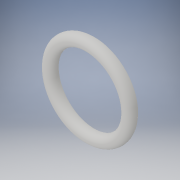
# Autodesk Inventor part: joint
Saved by Autodesk Inventor 2019 (Build 230136000, 136)
## iProperties
Created: 2018-04-17
Part Number: joint
Material: Générique
Document SubType Name: Modeling
Designer: Theo
Density: 1 g/cm^3
Appearance: Par défaut
Author: Theo
Autodesk Inventor part; units mm, degrees
ref_plane "YZ Plane" through (0, 0, 0) normal (1, 0, 0) x (0, 1, 0)
ref_plane "XZ Plane" through (0, 0, 0) normal (0, 1, 0) x (-1, 0, 0)
ref_plane "XY Plane" through (0, 0, 0) normal (0, 0, 1) x (1, 0, 0)
sketch "Esquisse1" plane through (0, 0, 0) normal (1, 0, 0) x (0, 1, 0)
  circle A0 centre (10, -1.5) radius 1.5
  line L0 (8.5, -0.5557) -> (8.5, -2.4443) construction
  line L1 (0, -3.6) -> (0, 0.6) projected
  line L2 (-2.3, 0) -> (13.8, 0) projected
  point P0 (0, 0)
  point P1 (8.5, -1.5)
  dimension "d0" = 3
  dimension "d1" = 8.5
  constraints: 2 end point, 2 horizontal alignment, 1 horizontal, 1 midpoint, 1 vertical, 2 other
  measures "d1" distance from line of point (0, 0) L0
revolve "Révolution1" add sketch "Esquisse1" angle 360 about axis through (0, 0, -10) along (0, 0, 1)
